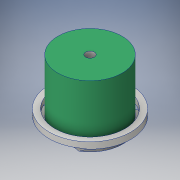
# Autodesk Inventor part: BrushlessInner
Saved by Autodesk Inventor 2016 (Build 200138000, 138)
## iProperties
Created: 2016-02-03
Part Number: BrushlessInner
Material: Generic
Document SubType Name: Modeling
Designer: Willis
Density: 1 g/cm^3
Appearance: Aluminum - Flat
Author: Willis
Autodesk Inventor part; units mm, degrees
ref_plane "YZ Plane" through (0, 0, 0) normal (1, 0, 0) x (0, 1, 0)
ref_plane "XZ Plane" through (0, 0, 0) normal (0, 1, 0) x (-1, 0, 0)
ref_plane "XY Plane" through (0, 0, 0) normal (0, 0, 1) x (1, 0, 0)
sketch "Sketch1" plane through (0, 0, 0) normal (0, 1, 0) x (-1, 0, 0)
  circle A0 centre (0, 0) radius 14
  circle A1 centre (0, 0) radius 12
  dimension "d0" = 28
  dimension "d1" = 2
  constraints: 2 centre point, 2 coincident
  measures "d0" diameter of A0
  measures "d1" radial gap between concentric circles of A0 A1
extrude "Extrusion1" add sketch "Sketch1" along normal blind 2
sketch "Sketch2" plane through (0, 0, 0) normal (0, -1, 0) x (1, 0, 0)
  line L0 (0, 0) -> (0, -37) construction
  arc A0 (9.1985, -10.5541) -> (-9.1985, -10.5541) centre (0, -37) ccw
  line L1 (0, 0) -> (0, 37) construction
  arc A1 (-9.1985, 10.5541) -> (9.1985, 10.5541) centre (0, 37) ccw
  line L2 (-13.0767, 5) -> (-9.0767, 5)
  line L3 (-9.0767, 5) -> (-9.0767, -5)
  line L4 (-9.0767, -5) -> (-13.0767, -5)
  line L5 (-7.8662, 0) -> (-7.8662, -5) construction
  arc A2 (9.1985, -10.5541) -> (9.1985, 10.5541) centre (0, 0) ccw
  arc A3 (-9.1985, 10.5541) -> (-13.0767, 5) centre (0, 0) ccw
  arc A4 (-13.0767, -5) -> (-9.1985, -10.5541) centre (0, 0) ccw
  line L6 (0, 0) -> (-9.0767, 0)
  dimension "d8" = 56
  dimension "d10" = 37
  dimension "d11" = 5
  dimension "d12" = 4
  constraints: 14 end point, 10 point on circle, 5 centre point, 3 coincident, 3 perpendicular, 2 equal length, 2 horizontal, 2 point on line, 2 vertical, 1 equal radius, 1 midpoint
  measures "d8" diameter of A0
  measures "d10" distance of L0.start L0.end
  measures "d11" distance of L5.start L5.end
  measures "d12" distance from line of L2.start L3
extrude "Extrusion2" add sketch "Sketch2" along normal blind 3
sketch "Sketch3" plane through (0, -3, 0) normal (0, -1, 0) x (1, 0, 0)
  circle A0 centre (0, 0) radius 1.5
  dimension "d15" = 3
  constraints: 1 centre point, 1 coincident
  measures "d15" diameter of A0
extrude "Extrusion3" cut sketch "Sketch3" against normal through all
chamfer "Chamfer1" distance 2.8 angle 45 3 edges at (-11.4786, -3, -8.0151) (-11.4786, -3, 8.0151) (14, -3, 0)
sketch "Sketch4" plane through (0, 0, 0) normal (0, 1, 0) x (1, 0, 0)
  circle A0 centre (0, 0) radius 1.5
  circle A1 centre (0, 0) radius 11
  dimension "d21" = 22
  dimension "d22" = 3
  constraints: 2 centre point, 2 coincident
  measures "d21" diameter of A1
  measures "d22" diameter of A0
extrude "Extrusion4" add sketch "Sketch4" along normal blind 18
sketch3d "Sketch6"
  constraints: 6 end point, 4 centre point, 4 coincident, 3 equal radius, 2 midpoint, 1 horizontal, 1 perpendicular
sketch " Sketch6" plane through (0, -3, 0) normal (0, -1, 0) x (1, 0, 0)
  line L0 (-6.7175, 6.7175) -> (6.7175, -6.7175) construction
  line L1 (5.6569, 5.6569) -> (-5.6569, -5.6569) construction
  circle A0 centre (-5.6569, -5.6569) radius 1.15
  circle A1 centre (6.7175, -6.7175) radius 1.15
  circle A2 centre (-6.7175, 6.7175) radius 1.15
  circle A3 centre (5.6569, 5.6569) radius 1.15
  circle A4 centre (0, 0) radius 1.5 construction
  line L2 (0, 0) -> (31.4092, 0) construction
extrude "Extrusion5" cut sketch " Sketch6" against normal up to surface (3 mm away)
body "Solid1"
